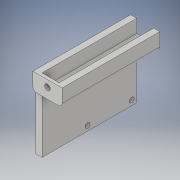
# Autodesk Inventor part: Yaw Motor Mount
Saved by Autodesk Inventor 2019 (Build 230136000, 136)
## iProperties
Created: 2018-05-28
Part Number: Yaw Motor Mount
Material: Generic
Document SubType Name: Modeling
Designer: samps
Density: 1 g/cm^3
Appearance: Default
Author: samps
Autodesk Inventor part; units mm, degrees
ref_plane "YZ Plane" through (0, 0, 0) normal (1, 0, 0) x (0, 1, 0)
ref_plane "XZ Plane" through (0, 0, 0) normal (0, 1, 0) x (-1, 0, 0)
ref_plane "XY Plane" through (0, 0, 0) normal (0, 0, 1) x (1, 0, 0)
sketch "Sketch1" plane through (0, 0, 0) normal (0, 0, 1) x (1, 0, 0)
  line L0 (0, 0) -> (0, -38.05)
  line L1 (0, -38.05) -> (3.175, -38.05)
  line L2 (3.175, -38.05) -> (3.175, 0)
  line L3 (3.175, 0) -> (0, 0)
  line L4 (3.175, 0) -> (3.175, -6.85)
  line L5 (3.175, -6.85) -> (12.025, -6.85)
  line L6 (12.025, -6.85) -> (12.025, 0)
  line L7 (12.025, 0) -> (15.2, 0)
  line L8 (15.2, 0) -> (15.2, -6.85)
  line L9 (15.2, -6.85) -> (15.2, -8.85)
  line L10 (15.2, -8.85) -> (3.175, -8.85)
  line L11 (0, -38.05) -> (0, -31.2)
  dimension "d0" = 38.05
  dimension "d1" = 3.175
  dimension "d2" = 6.85
  dimension "d3" = 8.85
  dimension "d4" = 3.175
  dimension "d5" = 2
  constraints: 24 end point, 7 perpendicular, 7 point on line, 1 vertical
  measures "d0" distance of L0.start L0.end
  measures "d1" distance of L0.end L1.end
  measures "d2" distance of L2.end L4.end
  measures "d3" distance of L4.end L5.end
  measures "d4" distance of L6.end L7.end
  measures "d5" distance of L8.end L9.end
extrude "Extrusion1" add sketch "Sketch1" along normal blind 49.213
sketch "Sketch2" plane through (0, 0, 0) normal (0, 0, -1) x (-1, 0, 0)
  line L0 (0, -38.05) -> (-3.175, -38.05) projected
  line L1 (0, -38.05) -> (0, -32.05)
  line L2 (0, 0) -> (0, -38.05) projected
  line L3 (0, -32.05) -> (0, -23.25)
  line L4 (0, -23.25) -> (6.6, -23.25)
  line L5 (6.6, -23.25) -> (6.6, -32.05)
  line L6 (6.6, -32.05) -> (0, -32.05)
  dimension "d12" = 6
  dimension "d13" = 8.8
  dimension "d14" = 6.6
  constraints: 10 end point, 3 perpendicular, 2 point on line
  measures "d12" distance of L0.start L1.end
  measures "d13" distance of L1.end L3.end
  measures "d14" distance of L3.end L4.end
extrude "Extrusion2" add sketch "Sketch2" against normal blind 3.175
sketch "Sketch3" plane through (0, 0, 3.175) normal (0, 0, 1) x (1, 0, 0)
  line L0 (0, -23.25) -> (0, -32.05) projected
  line L1 (0, -23.25) -> (-3.3, -23.25)
  line L2 (0, -23.25) -> (-6.6, -23.25) projected
  line L3 (-3.3, -23.25) -> (-3.3, -27.65)
  point P0 (0, 0)
  dimension "d17" = 4.4
  constraints: 4 end point, 1 midpoint, 1 vertical
  measures "d17" distance of L1.end L3.end
hole "Hole1" at (-3.3, -27.65, 3.175) direction (0, 0, -1) diameter 3 end through all
fillet "Fillet1" radius 2 2 edges at (-6.6, -23.25, 1.5875) (-6.6, -32.05, 1.5875)
sketch "Sketch4" plane through (0, 0, 49.213) normal (0, 0, 1) x (1, 0, 0)
  line L0 (3.175, 0) -> (0, 0) projected
  line L1 (3.175, -8.85) -> (15.2, -8.85) projected
  line L2 (0, 0) -> (15.2, 0)
  line L3 (15.2, 0) -> (15.2, -8.85)
  line L4 (15.2, -8.85) -> (0, -8.85)
  line L5 (0, -8.85) -> (0, 0)
  constraints: 8 end point, 2 parallel, 1 horizontal, 1 perpendicular
extrude "Extrusion3" add sketch "Sketch4" along normal blind 1.5875
sketch "Sketch5" plane through (0, 0, 50.8005) normal (0, 0, 1) x (1, 0, 0)
  line L0 (3.175, 0) -> (0, 0) projected
  line L1 (0, 0) -> (3.175, 0)
  line L2 (3.175, 0) -> (12.025, 0) projected
  line L3 (3.175, 0) -> (7.6, 0)
  line L4 (7.6, 0) -> (7.6, -3.425)
  dimension "d28" = 3.425
  constraints: 6 end point, 1 collinear, 1 midpoint, 1 vertical
  measures "d28" distance of L3.end L4.end
hole "Hole2" at (7.6, -3.425, 50.8005) direction (0, 0, -1) diameter 3 end through all
fillet "Fillet2" radius 2 2 edges at (0, -8.85, 50.0068) (15.2, -8.85, 25.4003)
sketch "Sketch6" plane through (0, -38.05, 0) normal (-1, 0, 0) x (0, 0, 1)
  line L0 (0, 0) -> (0, 29.2) projected
  line L1 (0, 0) -> (0, 28.2)
  line L2 (0, 28.2) -> (28.2, 28.2)
  line L3 (28.2, 28.2) -> (28.2, 0)
  line L4 (0, 0) -> (49.213, 0) projected
  line L5 (0, 0) -> (0, 14.1)
  line L6 (0, 12.8) -> (0, 14.8) projected
  line L7 (0, 14.1) -> (14.1, 14.1)
  line L8 (14.1, 14.1) -> (2.6, 14.1)
  line L9 (2.6, 14.1) -> (2.6, 2.6)
  line L10 (0, 12.8) -> (3.175, 12.8) projected
  line L11 (2.6, 2.6) -> (25.6, 2.6)
  line L12 (25.6, 2.6) -> (25.6, 25.6)
  line L13 (25.6, 25.6) -> (2.6, 25.6)
  line L14 (2.6, 25.6) -> (2.6, 2.6)
  point P0 (0, 38.05)
  dimension "d37" = 28.2
  dimension "d38" = 28.2
  dimension "d39" = 11.5
  dimension "d40" = 11.5
  dimension "d41" = 90
  dimension "d42" = 23
  dimension "d43" = 23
  constraints: 22 end point, 4 perpendicular, 4 point on line, 2 horizontal, 2 parallel
  measures "d37" distance of L0.start L1.end
  measures "d38" distance of L1.end L2.end
  measures "d39" distance of L7.end L8.end
  measures "d40" distance of L8.end L9.end
  measures "d41" angle of L9 L8
  measures "d42" distance of L13.end L12.end
  measures "d43" distance of L12.end L11.end
hole "Hole3" at (0, -35.45, 2.6) at (0, -35.45, 25.6) at (0, -12.45, 25.6) at (0, -12.45, 2.6) direction (1, 0, 0) diameter 2.5 end through all
body "Solid1"
